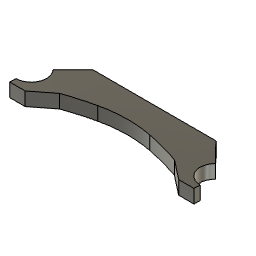
Finger1Section2P1V1 v2 (Autodesk Fusion 360 design; units mm, degrees)
Autodesk Fusion 360 part; units mm, degrees
sketch "Sketch1" plane through (0, 0, 0) normal (0, 0, 1) x (1, 0, 0)
  line L0 (4.507, 4) -> (5.507, 5)
  line L1 (2.2748, 1.7678) -> (4.507, 4)
  line L2 (0.507, -2.5) -> (0.507, -3.5)
  arc A0 (0.507, -2.5) -> (2.2748, 1.7678) centre (0.507, 0) ccw
  line L3 (0.507, -3.5) -> (3.007, -3.5)
  line L4 (3.007, -3.5) -> (6.1611, -1.04)
  line L5 (5.507, 5) -> (15.5594, 5)
  line L6 (25.5594, 5) -> (25.6118, 5)
  arc A1 (10.9966, 0.3532) -> (6.1611, -1.04) centre (20.507, -41.7412) ccw
  line L7 (15.5594, 5) -> (25.6118, 5)
  line L8 (25.6118, 5) -> (26.507, 4)
  arc A2 (24.8529, -1.04) -> (19.3514, 0.4515) centre (10.8341, -41.855) ccw
  line L9 (28.007, -3.5) -> (24.8529, -1.04)
  line L10 (30.507, -3.5) -> (28.007, -3.5)
  line L11 (30.507, -2.5) -> (30.507, -3.5)
  line L12 (15.5594, 1.1297) -> (15.5594, 1.0409)
  arc A3 (28.7392, 1.7678) -> (30.507, -2.5) centre (30.507, 0) ccw
  line L13 (28.7392, 1.7678) -> (26.507, 4)
  arc A4 (19.3514, 0.4515) -> (10.9966, 0.3532) centre (15.4041, -19.1551) ccw
  dimension "d12" = 5
  dimension "d16" = 2.5
  dimension "d17" = 4
  dimension "d30" = 5
  dimension "d31" = 2.5
  dimension "d32" = 4
  dimension "d33" = 20
  constraint perpendicular L2 L3
  constraint coincident L6.start L5
  constraint collinear L5 L6
  constraint perpendicular L10 L11
  constraint coincident L12.start A1
  constraint coincident L12.end A2
  constraint tangent A1 A4
  constraint tangent A2 A4
  measures "d12" diameter of A0
  measures "d16" distance of L2.end L3.end
  measures "d17" distance of L3.end L4.end
  measures "d30" diameter of A3
  measures "d31" distance of L10.start L9.start
  measures "d32" distance of L9.start A2.start
  measures "d33" radius of A4
extrude "Extrude2" add sketch "Sketch1" along normal blind 2.2
